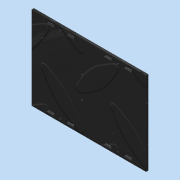
# Autodesk Inventor part: Box Bottom
Saved by Autodesk Inventor 2013 (Build 170138000, 138)
## iProperties
Created: 2012-12-29
Part Number: Box Bottom
Material: Generic
Document SubType Name: Modeling
Designer: Administrator
Density: 1 g/cm^3
Author: Administrator
Autodesk Inventor part; units mm, degrees
ref_plane "YZ Plane" through (0, 0, 0) normal (1, 0, 0) x (0, 1, 0)
ref_plane "XZ Plane" through (0, 0, 0) normal (0, 1, 0) x (-1, 0, 0)
ref_plane "XY Plane" through (0, 0, 0) normal (0, 0, 1) x (1, 0, 0)
sketch "Sketch1" plane through (0, 0, 0) normal (0, 0, 1) x (1, 0, 0)
  line L0 (74.217, 53.2739) -> (74.217, -53.4061)
  line L1 (-72.183, -53.4061) -> (-72.183, 53.2739)
  line L2 (36.8493, 53.2398) -> (36.8645, 53.2398)
  line L3 (74.217, -53.4061) -> (39.2667, -53.4061)
  circle A0 centre (-35.6832, 48.84) radius 1.525
  circle A1 centre (37.7209, 48.84) radius 1.525
  line L4 (39.2667, -53.4061) -> (-72.183, -53.4061)
  circle A2 centre (-35.6832, -48.9061) radius 1.525
  circle A3 centre (37.7172, -48.9061) radius 1.525
  circle A4 centre (-58.6221, 29.2099) radius 1.6
  circle A5 centre (-7.8221, 13.9699) radius 1.6
  circle A6 centre (-7.8221, -13.9701) radius 1.6
  line L5 (-43.5082, -47.3313) -> (-53.6082, -47.3313)
  line L6 (-53.6082, -47.3313) -> (-53.6082, -50.4313)
  line L7 (-53.6082, -50.4313) -> (-43.5082, -50.4313)
  line L8 (-43.5082, -50.4313) -> (-43.5082, -47.3313)
  line L9 (-27.8582, -47.3199) -> (-17.7582, -47.3199)
  line L10 (-17.7582, -47.3199) -> (-17.7582, -50.4199)
  line L11 (-17.7582, -50.4199) -> (-27.8582, -50.4199)
  line L12 (-27.8582, -50.4199) -> (-27.8582, -47.3199)
  line L13 (29.8922, -47.3706) -> (19.7922, -47.3706)
  line L14 (19.7922, -47.3706) -> (19.7922, -50.4706)
  line L15 (19.7922, -50.4706) -> (29.8922, -50.4706)
  line L16 (29.8922, -50.4706) -> (29.8922, -47.3706)
  line L17 (45.5422, -47.3706) -> (55.6422, -47.3706)
  line L18 (55.6422, -47.3706) -> (55.6422, -50.4706)
  line L19 (55.6422, -50.4706) -> (45.5422, -50.4706)
  line L20 (45.5422, -50.4706) -> (45.5422, -47.3706)
  line L21 (-72.183, 53.2739) -> (74.217, 53.2739)
  line L22 (45.5459, 50.3571) -> (55.6459, 50.3571)
  line L23 (55.6459, 50.3571) -> (55.6459, 47.2571)
  line L24 (55.6459, 47.2571) -> (45.5459, 47.2571)
  line L25 (45.5459, 47.2571) -> (45.5459, 50.3571)
  line L26 (29.8959, 50.3571) -> (19.7959, 50.3571)
  line L27 (19.7959, 50.3571) -> (19.7959, 47.2571)
  line L28 (19.7959, 47.2571) -> (29.8959, 47.2571)
  line L29 (29.8959, 47.2571) -> (29.8959, 50.3571)
  line L30 (-43.5082, 50.3529) -> (-53.6082, 50.3529)
  line L31 (-53.6082, 50.3529) -> (-53.6082, 47.2529)
  line L32 (-53.6082, 47.2529) -> (-43.5082, 47.2529)
  line L33 (-43.5082, 47.2529) -> (-43.5082, 50.3529)
  line L34 (-27.8582, 50.3571) -> (-17.7582, 50.3571)
  line L35 (-17.7582, 50.3571) -> (-17.7582, 47.2571)
  line L36 (-17.7582, 47.2571) -> (-27.8582, 47.2571)
  line L37 (-27.8582, 47.2571) -> (-27.8582, 50.3571)
  point P0 (0, 0)
  dimension "d0" = 146.4
  dimension "d1" = 106.68
  dimension "d43" = 3.05
  dimension "d47" = 3.05
  dimension "d48" = 36.4961
  dimension "d50" = 3.05
  dimension "d52" = 36.4998
  dimension "d53" = 3.05
  dimension "d54" = 36.4998
  dimension "d60" = 3.2
  dimension "d63" = 3.2
  dimension "d66" = 3.2
  dimension "d69" = 27.94
  dimension "d70" = 53.0368
  dimension "d73" = 10.1
  dimension "d74" = 3.1
  dimension "d76" = 10.1
  dimension "d77" = 3.1
  dimension "d79" = 10.1
  dimension "d80" = 3.1
  dimension "d81" = 10.1
  dimension "d82" = 3.1
  dimension "d85" = 10.1
  dimension "d86" = 3.1
  dimension "d87" = 10.1
  dimension "d88" = 3.1
  dimension "d91" = 10.1
  dimension "d92" = 3.1
  dimension "d93" = 10.1
  dimension "d94" = 3.1
  dimension "d99" = 6.3
  dimension "d100" = 6.3
  dimension "d101" = 6.3
  dimension "d102" = 6.3
  dimension "d103" = 6.3
  dimension "d104" = 6.3
  dimension "d105" = 6.3
  dimension "d106" = 6.3
  dimension "d107" = 2.9168
  dimension "d108" = 2.921
  dimension "d109" = 2.9168
  dimension "d110" = 2.9168
  dimension "d111" = 2.9355
  dimension "d112" = 2.9355
  constraints: 76 end point, 18 parallel, 10 perpendicular, 9 horizontal, 7 centre point, 1 collinear
  measures "d0" distance of L0.end L1.start
  measures "d1" distance of L0.start L0.end
  measures "d43" diameter of A0
  measures "d47" diameter of A1
  measures "d48" distance from line of L0 A1.centre
  measures "d50" diameter of A2
  measures "d52" distance from line of L1 A2.centre
  measures "d53" diameter of A3
  measures "d54" distance from line of L0 A3.centre
  measures "d60" diameter of A4
  measures "d63" diameter of A5
  measures "d66" diameter of A6
  measures "d69" distance of A6.centre A5.centre
  measures "d70" distance of A4.centre A5.centre
  measures "d73" distance of L7.end L6.end
  measures "d74" distance of L6.end L5.end
  measures "d76" distance of L10.end L11.end
  measures "d77" distance of L9.end L10.end
  measures "d79" distance of L15.end L14.end
  measures "d80" distance of L14.end L13.end
  measures "d81" distance of L18.end L19.end
  measures "d82" distance of L17.end L18.end
  measures "d85" distance of L23.end L24.end
  measures "d86" distance of L22.end L23.end
  measures "d87" distance of L28.end L27.end
  measures "d88" distance of L27.end L26.end
  measures "d91" distance of L32.end L31.end
  measures "d92" distance of L31.end L30.end
  measures "d93" distance of L35.end L36.end
  measures "d94" distance of L34.end L35.end
  measures "d99" distance edge to line of A2 L8
  measures "d100" distance edge to line of A2 L12
  measures "d101" distance edge to line of A3 L16
  measures "d102" distance edge to line of A3 L20
  measures "d103" distance edge to line of A1 L29
  measures "d104" distance edge to line of A1 L25
  measures "d105" distance edge to line of A0 L37
  measures "d106" distance edge to line of A0 L33
  measures "d107" distance between parallel lines of L34 L21
  measures "d108" distance between parallel lines of L21 L30
  measures "d109" distance between parallel lines of L26 L21
  measures "d110" distance between parallel lines of L22 L21
  measures "d111" distance between parallel lines of L3 L19
  measures "d112" distance between parallel lines of L4 L15
extrude "Extrusion4" add sketch "Sketch1" along normal blind 3
body "Solid4"
